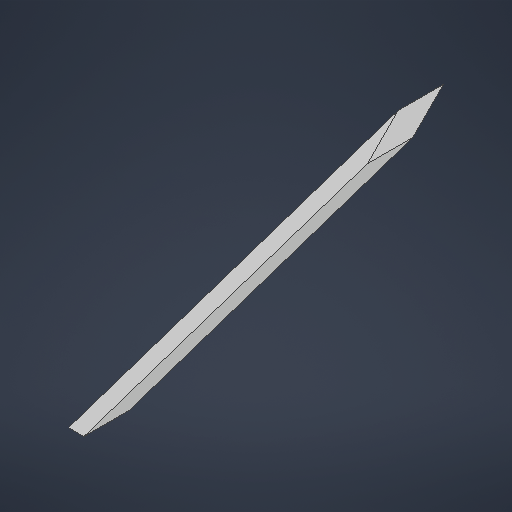
# Autodesk Inventor part: SS_2x4x36
Saved by Autodesk Inventor 2026 (Build 300175000, 175)
## iProperties
Created: 2025-09-04
Part Number: SS_2x4x36
Material: Generic
Document SubType Name: Modeling
Designer: trott
Density: 1 g/cm^3
Appearance: Default
Author: trott
Autodesk Inventor part; units mm, degrees
ref_plane "YZ Plane" through (0, 0, 0) normal (1, 0, 0) x (0, 1, 0)
ref_plane "XZ Plane" through (0, 0, 0) normal (0, 1, 0) x (-1, 0, 0)
ref_plane "XY Plane" through (0, 0, 0) normal (0, 0, 1) x (1, 0, 0)
sketch "Sketch2" plane through (0, 0, 0) normal (0, 0, 1) x (1, 0, 0)
  line L0 (0, 0) -> (0, 609.6)
  line L1 (0, 0) -> (-304.8, 0)
  line L2 (-304.8, 0) -> (0, 609.6)
  line L3 (-304.8, 0) -> (-270.7223, -17.0388)
  line L4 (0, 609.6) -> (34.0777, 592.5612)
  line L5 (-270.7223, -17.0388) -> (34.0777, 592.5612)
  line L6 (0, 609.6) -> (-304.8, 609.6)
  line L7 (-304.8, 609.6) -> (-304.8, 0)
  point P0 (0, 524.4058)
  point P1 (-262.2029, 0)
  dimension "d4" = 609.6
  dimension "d5" = 304.8
  dimension "d6" = 38.1
  dimension "d7" = 38.1
  dimension "d13" = 304.8
  constraints: 16 end point, 2 horizontal, 2 perpendicular, 1 vertical
  measures "d4" distance of L0.start L0.end
  measures "d5" distance of L0.start L1.end
  measures "d6" distance of L1.end L3.end
  measures "d7" distance of L0.end L4.end
  measures "d13" distance of L0.end L6.end
sketch "Sketch3" plane through (0, 0, 0) normal (1, 0, 0) x (0, 1, 0)
  line L0 (0, 0) -> (0, 609.6)
  line L1 (0, 0) -> (609.6, 0)
  line L2 (609.6, 0) -> (0, 609.6)
  line L3 (0, 609.6) -> (-62.8618, 546.7382)
  line L4 (-62.8618, 546.7382) -> (546.7382, -62.8618)
  line L5 (609.6, 0) -> (609.6, -304.8)
  line L6 (546.7382, -62.8618) -> (609.6, -125.7236)
  point P0 (0, 483.8764)
  point P1 (483.8764, 0)
  dimension "d8" = 609.6
  dimension "d9" = 609.6
  dimension "d10" = 88.9
  dimension "d16" = 304.8
  constraints: 14 end point, 2 vertical, 1 horizontal, 1 parallel, 1 perpendicular, 1 point on line
  measures "d8" distance of L0.start L0.end
  measures "d9" distance of L0.start L1.end
  measures "d10" distance of L0.end L3.end
  measures "d16" distance of L1.end L5.end
extrude "Extrusion2" add sketch "Sketch3" against normal blind 304.8 contours L0 L2 L1 L4 | L1 L5 L6 L4
extrude "Extrusion3" cut sketch "Sketch2" along normal mid plane 1219.2 contours L1 L5 L0 | L2 L7 L6
body "Solid2"
